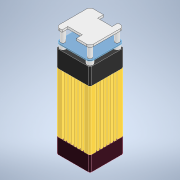
# Autodesk Inventor part: 13_Lasermodule_10W
Saved by Autodesk Inventor 2022.2 (Build 262287010, 287A)
## iProperties
Created: 2022-03-20
Part Number: 13_Lasermodule_10W
Material: ABS-Kunststoff
Document SubType Name: Modeling
Designer: MXBD
Density: 1.06 g/cm^3
Appearance: Glatt - Weiß
Author: MXBD
Autodesk Inventor part; units mm, degrees
ref_plane "YZ Plane" through (0, 0, 0) normal (1, 0, 0) x (0, 1, 0)
sketch "Skizze1" plane through (0, 0, 0) normal (0, 1, 0) x (-1, 0, 0)
  line L0 (20, 20) -> (-20, 20)
  line L1 (-20, 20) -> (-20, -20)
  line L2 (-20, -20) -> (20, -20)
  line L3 (20, -20) -> (20, 20)
  line L4 (20, 20) -> (-20, -20) construction
  line L5 (-20, 20) -> (20, -20) construction
  point P0 (0, 0)
  dimension "d0" = 40
  dimension "d1" = 40
  constraints: 12 end point, 2 midpoint, 2 parallel, 1 horizontal, 1 perpendicular
  measures "d0" distance of L2.end L1.end
  measures "d1" distance of L1.end L0.end
extrude "Extrusion1" add sketch "Skizze1" along normal blind 18
sketch "Skizze2" plane through (0, 18, 0) normal (0, 1, 0) x (1, 0, 0)
  line L0 (20, 20) -> (-20, 20) projected
  line L1 (20, -20) -> (-20, -20)
  line L2 (-20, -20) -> (-20, 20)
  line L3 (-20, 20) -> (20, 20)
  line L4 (20, 20) -> (20, -20)
  line L5 (20, -20) -> (-20, 20) construction
  line L6 (-20, -20) -> (20, 20) construction
  point P0 (0, 0)
  constraints: 12 end point, 2 midpoint, 2 parallel, 1 horizontal, 1 perpendicular
extrude "Extrusion2" add sketch "Skizze2" along normal blind 70 separate body
sketch "Skizze3" plane through (0, 88, 0) normal (0, 1, 0) x (1, 0, 0)
  line L0 (20, 20) -> (-20, 20) projected
  line L1 (20, -20) -> (-20, -20)
  line L2 (-20, -20) -> (-20, 20)
  line L3 (-20, 20) -> (20, 20)
  line L4 (20, 20) -> (20, -20)
  line L5 (20, -20) -> (-20, 20) construction
  line L6 (-20, -20) -> (20, 20) construction
  point P0 (0, 0)
  constraints: 12 end point, 2 midpoint, 2 parallel, 1 horizontal, 1 perpendicular
extrude "Extrusion3" add sketch "Skizze3" along normal blind 20 separate body
fillet "Rundung1" radius 2 4 edges at (20, 98, 20) (20, 98, -20) (-20, 98, 20) (-20, 98, -20)
sketch "Skizze4" plane through (0, 108, 0) normal (0, 1, 0) x (1, 0, 0)
  line L0 (16, -16) -> (-16, -16) construction
  line L1 (-16, -16) -> (-16, 16) construction
  line L2 (-16, 16) -> (16, 16) construction
  line L3 (16, 16) -> (16, -16) construction
  line L4 (16, -16) -> (-16, 16) construction
  line L5 (-16, -16) -> (16, 16) construction
  circle A0 centre (-16, -16) radius 3.5
  circle A1 centre (-16, 16) radius 3.5
  circle A2 centre (16, 16) radius 3.5
  circle A3 centre (16, -16) radius 3.5
  point P0 (0, 0)
  dimension "d9" = 32
  dimension "d10" = 32
  dimension "d11" = 7
  constraints: 12 end point, 4 centre point, 4 coincident, 3 equal radius, 2 midpoint, 2 parallel, 1 horizontal, 1 perpendicular
  measures "d9" distance of L1.end L2.end
  measures "d10" distance of L0.end L1.end
  measures "d11" diameter of A0
extrude "Extrusion4" add sketch "Skizze4" along normal blind 5 separate body
ref_plane "Arbeitsebene1" through (0, 113, 0) normal (0, 1, 0) x (1, 0, 0)
sketch "Skizze5" plane through (0, 113, 0) normal (0, 1, 0) x (1, 0, 0)
  line L0 (20, 20) -> (-20, 20) projected
  line L1 (20, -20) -> (-20, -20)
  line L2 (-20, -20) -> (-20, 20)
  line L3 (-20, 20) -> (20, 20)
  line L4 (20, 20) -> (20, -20)
  line L5 (20, -20) -> (-20, 20) construction
  line L6 (-20, -20) -> (20, 20) construction
  point P0 (0, 0)
  constraints: 12 end point, 2 midpoint, 2 parallel, 1 horizontal, 1 perpendicular
extrude "Extrusion5" add sketch "Skizze5" along normal blind 1.5 separate body
sketch "Skizze6" plane through (0, 114.5, 0) normal (0, 1, 0) x (1, 0, 0)
  circle A0 centre (16, 16) radius 3.5 construction
  line L0 (-16, -16) -> (16, -16) construction
  line L1 (16, -16) -> (16, 16) construction
  line L2 (16, 16) -> (-16, 16) construction
  line L3 (-16, 16) -> (-16, -16) construction
  line L4 (-16, -16) -> (16, 16) construction
  line L5 (16, -16) -> (-16, 16) construction
  circle A1 centre (16, 16) radius 2.5
  circle A2 centre (-16, 16) radius 2.5
  circle A3 centre (-16, -16) radius 2.5
  circle A4 centre (16, -16) radius 3.5 projected
  circle A5 centre (16, -16) radius 2.5
  point P0 (0, 0)
  dimension "d17" = 5
  constraints: 12 end point, 4 centre point, 4 coincident, 3 equal radius, 2 midpoint, 2 parallel, 1 horizontal, 1 perpendicular
  measures "d17" diameter of A1
extrude "Extrusion6" add sketch "Skizze6" along normal blind 12.7 separate body contours A1 | A2 | A3 | A5
ref_plane "Arbeitsebene2" through (0, 127.2, 0) normal (0, 1, 0) x (1, 0, 0)
sketch "Skizze7" plane through (0, 127.2, 0) normal (0, 1, 0) x (1, 0, 0)
  line L0 (-20, -20) -> (20, -20)
  line L1 (20, -20) -> (20, 20)
  line L2 (20, 20) -> (-20, 20)
  line L3 (-20, 20) -> (-20, -20)
  line L4 (-20, -20) -> (20, 20) construction
  line L5 (20, -20) -> (-20, 20) construction
  point P0 (0, 0)
  dimension "d21" = 40
  dimension "d22" = 40
  constraints: 12 end point, 2 midpoint, 2 parallel, 1 horizontal, 1 perpendicular
  measures "d21" distance of L2.end L1.end
  measures "d22" distance of L1.end L0.end
extrude "Extrusion7" add sketch "Skizze7" along normal blind 2.5 separate body
sketch "Skizze8" plane through (0, 0, 0) normal (0, -1, 0) x (1, 0, 0)
  line L0 (-18, 18) -> (18, 18)
  line L1 (18, 18) -> (18, -18)
  line L2 (18, -18) -> (-18, -18)
  line L3 (-18, -18) -> (-18, 18)
  line L4 (-18, 18) -> (18, -18) construction
  line L5 (18, 18) -> (-18, -18) construction
  point P0 (0, 0)
  dimension "d25" = 36
  dimension "d26" = 36
  constraints: 12 end point, 2 midpoint, 2 parallel, 1 horizontal, 1 perpendicular
  measures "d25" distance of L1.end L2.end
  measures "d26" distance of L0.end L1.end
extrude "Extrusion8" cut sketch "Skizze8" against normal blind 16 bodies 1
sketch "Skizze9" plane through (-20, 0, -20) normal (-1, 0, 0) x (0, 0, 1)
  line L0 (0, 0) -> (40, 0) projected
  arc A0 (32, 0) -> (8, 0) centre (20, 0) ccw
  line L1 (8, 0) -> (32, 0)
  dimension "d29" = 12
  constraints: 2 end point, 2 point on circle, 1 centre point, 1 coincident, 1 horizontal, 1 point on line
  measures "d29" radius of A0
extrude "Extrusion9" cut sketch "Skizze9" against normal up to surface (2 mm away) bodies 1
sketch "Skizze10" plane through (0, 16, 0) normal (0, -1, 0) x (1, 0, 0)
  line L0 (0, 28) -> (0, -28) projected
  line L1 (-28, 0) -> (28, 0) projected
  line L2 (16, 0) -> (16, -12)
  line L3 (16, -12) -> (12, -16)
  line L4 (12, -16) -> (0, -16)
  line L5 (20, 20) -> (20, -20) projected
  line L6 (20, -20) -> (-20, -20) projected
  line L7 (16, 0) -> (16, 12)
  line L8 (16, 12) -> (12, 16)
  line L9 (12, 16) -> (0, 16)
  line L10 (-16, 0) -> (-16, -12)
  line L11 (-16, -12) -> (-12, -16)
  line L12 (-12, -16) -> (0, -16)
  line L13 (-16, 0) -> (-16, 12)
  line L14 (-16, 12) -> (-12, 16)
  line L15 (-12, 16) -> (0, 16)
  point P0 (0, 0)
  dimension "d32" = 4
  dimension "d34" = 8
  dimension "d36" = 8
  dimension "d37" = 4
  constraints: 24 end point, 8 symmetric about line, 2 point on line, 1 perpendicular, 1 vertical
  measures "d32" distance between parallel lines of L2 L5
  measures "d34" distance from line of L6 L2.end
  measures "d36" distance from line of L5 L3.end
  measures "d37" distance between parallel lines of L6 L4
extrude "Extrusion10" cut sketch "Skizze10" against normal blind 2 contours L9 L8 L7 L1 L0 | L0 L1 L13 L14 L15 | L1 L2 L3 L4 L0 | L0 L12 L11 L10 L1 bodies 1
sketch "Skizze11" plane through (0, 18, 0) normal (0, -1, 0) x (1, 0, 0)
  line L0 (20, 20) -> (20, -20) projected
  line L1 (-28, 0) -> (28, 0) projected
  line L2 (18, 1) -> (22, 1)
  line L3 (22, 1) -> (22, -1)
  line L4 (22, -1) -> (18, -1)
  line L5 (18, -1) -> (18, 1)
  line L6 (18, 1) -> (22, -1) construction
  line L7 (22, 1) -> (18, -1) construction
  point P0 (0, 0)
  point P1 (20, 0)
  point P2 (20, -1)
  point P3 (20, 1)
  dimension "d40" = 4
  dimension "d41" = 2
  constraints: 12 end point, 3 midpoint, 2 parallel, 1 horizontal, 1 perpendicular, 1 point on line
  measures "d40" distance of L3.end L4.end
  measures "d41" distance of L2.end L3.end
extrude "Extrusion11" cut sketch "Skizze11" against normal blind 70 contours L0 L1 L5 L2 | L0 L4 L5 L1 bodies 2
pattern_linear "Rechteckige Anordnung1" count 4 spacing 4 along (0, 0, -1) count 4 spacing 4 along (0, 0, 1) of "Extrusion11" bodies 2
sketch "Skizze12" plane through (0, 18, 0) normal (0, -1, 0) x (1, 0, 0)
  line L0 (0, 28) -> (0, -28) projected
  line L1 (-1, 22) -> (1, 22)
  line L2 (1, 22) -> (1, 18)
  line L3 (1, 18) -> (-1, 18)
  line L4 (-1, 18) -> (-1, 22)
  line L5 (-20, 20) -> (20, 20) projected
  line L6 (-1, 22) -> (1, 18) construction
  line L7 (1, 22) -> (-1, 18) construction
  point P0 (0, 0)
  point P1 (0, 20)
  point P2 (1, 20)
  point P3 (-1, 20)
  dimension "d50" = 2
  dimension "d51" = 4
  constraints: 12 end point, 3 midpoint, 2 parallel, 1 horizontal, 1 perpendicular
  measures "d50" distance of L2.end L3.end
  measures "d51" distance of L1.end L2.end
extrude "Extrusion12" cut sketch "Skizze12" against normal blind 70 contours L5 L2 L3 L0 | L0 L3 L4 L5 bodies 2
pattern_linear "Rechteckige Anordnung2" count 4 spacing 4 along (1, 0, 0) count 4 spacing 4 along (-1, 0, 0) of "Extrusion12" bodies 2
mirror "Spiegeln1" about plane through (0, 0, 0) normal (0, 0, 1) of "Extrusion12", "Rechteckige Anordnung2" bodies 2
fillet "Rundung2" radius 4 8 edges at (20, 113.75, 20) (-20, 113.75, 20) (-20, 113.75, -20) (20, 113.75, -20) (20, 128.45, 20) (-20, 128.45, 20) (-20, 128.45, -20) (20, 128.45, -20)
fillet "Rundung3" radius 2 8 edges at (20, 9, 20) (20, 9, -20) (-20, 9, -20) (-20, 9, 20) (20, 53, -20) (-20, 53, -20) (-20, 53, 20) (20, 53, 20)
fillet "Rundung4" radius 1 2 edges at (-19, 0, -12) (-19, 0, 12)
sketch "Skizze13" plane through (0, 129.7, 0) normal (0, 1, 0) x (1, 0, 0)
  line L0 (-18, -20) -> (18, -20) projected
  line L1 (-13, -20) -> (4, -20)
  line L2 (4, -20) -> (4, -13)
  line L3 (4, -13) -> (-13, -13)
  line L4 (-13, -13) -> (-13, -20)
  line L5 (18, 20) -> (-18, 20) projected
  line L6 (-4, 20) -> (13, 20)
  line L7 (13, 20) -> (13, 13)
  line L8 (13, 13) -> (-4, 13)
  line L9 (-4, 13) -> (-4, 20)
  line L10 (-20, 16) -> (-20, -16) projected
  line L11 (20, -16) -> (20, 16) projected
  point P0 (0, 0)
  point P1 (-4, 16.5)
  point P2 (4.5, 20)
  point P3 (4.5, 13)
  dimension "d63" = 7
  dimension "d64" = 17
  dimension "d65" = 7
  dimension "d66" = 17
  dimension "d67" = 7
  dimension "d68" = 7
  constraints: 16 end point, 4 parallel, 3 midpoint, 2 horizontal, 2 perpendicular, 2 point on line
  measures "d63" distance between parallel lines of L0 L3
  measures "d64" distance between parallel lines of L2 L4
  measures "d65" distance between parallel lines of L10 L4
  measures "d66" distance from line of L7 point (-4, 16.5)
  measures "d67" distance of point (4.5, 20) point (4.5, 13)
  measures "d68" distance between parallel lines of L11 L7
extrude "Extrusion13" cut sketch "Skizze13" against normal up to surface (2.5 mm away) bodies 7
sketch "Skizze14" plane through (-20, 18, -18) normal (-1, 0, 0) x (0, 0, 1)
  line L0 (18, 137.64) -> (18, -43.94) projected
  line L1 (0, 70) -> (36, 70) projected
  point P0 (18, -18)
  point P1 (18, 57)
  point P2 (18, 47)
  point P3 (18, 27)
  dimension "d71" = 10
  dimension "d72" = 20
  dimension "d73" = 13
  constraints: 3 point on line
  measures "d71" distance of point (18, 47) point (18, 57)
  measures "d72" distance of point (18, 27) point (18, 47)
  measures "d73" distance from line of L1 point (18, 57)
hole "Bohrung1" at (-20, 75, 0) at (-20, 65, 0) at (-20, 45, 0) direction (1, 0, 0) diameter 2.459 depth 8.8 tip angle 118 bodies 2 thread size "M3x0.5" class "6H" standard "ISO Metric profile"
sketch "Skizze15" plane through (-20, 18, -18) normal (-1, 0, 0) x (0, 0, 1)
  line L0 (18, 137.64) -> (18, -43.94) projected
  point P0 (18, -18)
  point P1 (26, 58.1092)
  point P2 (28, 53.1092)
  point P3 (10, 58.1092)
  point P4 (8, 53.1092)
  dimension "d81" = 5
  dimension "d82" = 10
  dimension "d83" = 8
  constraints: 2 symmetric about line
  measures "d81" vertical distance of point (28, 53.109) point (26, 58.109)
  measures "d82" distance from line of L0 point (28, 53.109)
  measures "d83" distance from line of L0 point (26, 58.109)
hole "Bohrung2" at (-20, 76.1092, 8) at (-20, 71.1092, 10) at (-20, 76.1092, -8) at (-20, 71.1092, -10) direction (1, 0, 0) diameter 2.459 depth 8.8 tip angle 118 bodies 2 thread size "M3x0.5" class "6H" standard "ISO Metric profile"
sketch "Skizze16" plane through (-20, 18, -18) normal (-1, 0, 0) x (0, 0, 1)
  line L0 (18, 137.64) -> (18, -43.94) projected
  circle A0 centre (18, 47) radius 1.2295 projected
  point P0 (18, -18)
  point P1 (18, 7)
  point P2 (26, 12)
  point P3 (28, 7)
  point P4 (10, 12)
  point P5 (8, 7)
  dimension "d91" = 40
  dimension "d92" = 10
  dimension "d93" = 8
  dimension "d94" = 5
  constraints: 2 symmetric about line, 1 horizontal alignment, 1 point on line
  measures "d91" distance of A0.centre point (18, 7)
  measures "d92" distance of point (28, 7) point (18, 7)
  measures "d93" horizontal distance of point (26, 12) point (18, 7)
  measures "d94" vertical distance of point (28, 7) point (26, 12)
hole "Bohrung3" at (-20, 25, 0) at (-20, 30, 8) at (-20, 25, 10) at (-20, 30, -8) at (-20, 25, -10) direction (1, 0, 0) diameter 2.459 depth 8.8 tip angle 118 bodies 2 thread size "M3x0.5" class "6H" standard "ISO Metric profile"
sketch "Skizze17" plane through (0, 18, 0) normal (0, -1, 0) x (1, 0, 0)
  circle A0 centre (0, 0) radius 4
  dimension "d102" = 8
  constraints: 1 centre point, 1 coincident
  measures "d102" diameter of A0
extrude "Extrusion14" cut sketch "Skizze17" against normal blind 1 bodies 2
equation "\"d9\" = d10"
equation "\"d26\" = d25"
equation "\"d36\" = d34"
equation "\"d37\" = d32"
equation "\"d66\" = d64"
equation "\"d67\" = d63"
equation "\"d68\" = d65"
